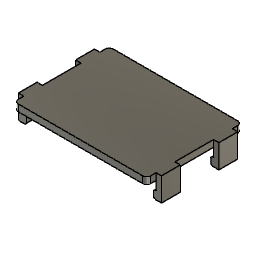
bluetooth module box (Autodesk Fusion 360 design; units mm, degrees)
Autodesk Fusion 360 part; units mm, degrees
note: some values were not read from the file. Set by a fixed rule: which sketch regions a step uses.
sketch "Sketch1" plane through (0, 0, 0) normal (0, 0, 1) x (1, 0, 0) in component "bottom"
  line L0 (0, 0) -> (49.2, 0)
  line L1 (49.2, 0) -> (49.2, 38.3)
  line L2 (49.2, 38.3) -> (0, 38.3)
  line L3 (0, 38.3) -> (0, 0)
  dimension "d6" = 38.3
  dimension "d7" = 49.2
  constraint horizontal L0
  constraint vertical L1
  constraint horizontal L2
  constraint vertical L3
  constraint coincident L0.start L3.end
  measures "d6" distance of L0.end L1.end
  measures "d7" distance of L1.end L2.end
extrude "Extrude1" add sketch "Sketch1" along normal blind 3 makes body 1 in component "bottom"
sketch "Sketch2" plane through (0, 0, 3) normal (0, 0, 1) x (-1, 0, 0) in component "bottom"
  line L0 (0, -38.3) -> (0, 0)
  line L1 (0, 0) -> (-49.2, 0)
  line L2 (-49.2, 0) -> (-49.2, -38.3)
  line L3 (-49.2, -38.3) -> (0, -38.3)
  line L4 (-46.2, -3) -> (-46.2, -35.3)
  line L5 (-46.2, -35.3) -> (-3, -35.3)
  line L6 (-3, -35.3) -> (-3, -3)
  line L7 (-3, -3) -> (-46.2, -3)
extrude "Extrude2" add sketch "Sketch2" along normal blind 12.2 bodies 1 in component "bottom"
sketch "Sketch3" plane through (0, 0, 0) normal (0, -1, 0) x (1, 0, 0) in component "bottom"
  line L0 (0, 0) -> (49.2, 0)
  line L1 (49.2, 0) -> (49.2, 15.2)
  line L2 (49.2, 15.2) -> (0, 15.2)
  line L3 (0, 15.2) -> (0, 0)
  line L4 (29.1, 10.2) -> (44.1, 10.2)
  line L5 (44.1, 10.2) -> (44.1, 7.2)
  line L6 (44.1, 7.2) -> (29.1, 7.2)
  line L7 (29.1, 7.2) -> (29.1, 10.2)
  line L8 (19.6, 12.2) -> (26.1, 12.2)
  line L9 (26.1, 12.2) -> (26.1, 7.2)
  line L10 (26.1, 7.2) -> (19.6, 7.2)
  line L11 (19.6, 7.2) -> (19.6, 12.2)
  line L12 (7.1, 10.2) -> (16.1, 10.2)
  line L13 (16.1, 10.2) -> (16.1, 7.2)
  line L14 (16.1, 7.2) -> (7.1, 7.2)
  line L15 (7.1, 7.2) -> (7.1, 10.2)
  dimension "d13" = 5.1
  dimension "d14" = 7.2
  dimension "d15" = 3
  dimension "d16" = 15
  dimension "d17" = 23.1
  dimension "d18" = 6.5
  dimension "d20" = 7.1
  dimension "d21" = 9
  dimension "d22" = 3
  dimension "d44" = 5
  constraint horizontal L4
  constraint vertical L5
  constraint horizontal L6
  constraint vertical L7
  constraint vertical L9
  constraint horizontal L10
  constraint vertical L11
  constraint collinear L6 L10
  constraint horizontal L12
  constraint vertical L13
  constraint horizontal L14
  constraint vertical L15
  constraint collinear L10 L14
  measures "d13" distance of L1 L5
  measures "d14" distance of L0 L6
  measures "d15" distance of L4.end L5.end
  measures "d16" distance of L4.start L4.end
  measures "d17" distance of L1 L9
  measures "d18" distance of L8.start L8.end
  measures "d20" distance of L3 L15
  measures "d21" distance of L12.start L12.end
  measures "d22" distance of L12.start L14.end
  measures "d44" distance of L8 L10
extrude "Extrude3" cut sketch "Sketch3" against normal blind 3 contours L4 L5 L6 L7 | L8 L9 L10 L11 | L12 L13 L14 L15 bodies 1 in component "bottom"
sketch "Sketch4" plane through (0, 0, 3) normal (0, 0, 1) x (-1, 0, 0) in component "bottom"
  line L0 (-46.2, -3) -> (-46.2, -35.3)
  line L1 (-46.2, -35.3) -> (-3, -35.3)
  line L2 (-3, -35.3) -> (-3, -3)
  line L3 (-3, -3) -> (-46.2, -3)
  line L4 (-5, -5) -> (-44.2, -5) construction
  line L5 (-44.2, -5) -> (-44.2, -33.3) construction
  line L6 (-44.2, -33.3) -> (-5, -33.3) construction
  line L7 (-5, -33.3) -> (-5, -5) construction
  circle A0 centre (-5, -33.3) radius 2
  circle A1 centre (-44.2, -33.3) radius 2
  circle A2 centre (-44.2, -5) radius 2
  circle A3 centre (-5, -5) radius 2
  line L8 (-3, -6) -> (-46.2, -6)
  line L9 (-46.2, -6) -> (-46.2, -3)
  line L10 (-46.2, -3) -> (-3, -3)
  line L11 (-3, -3) -> (-3, -6)
  dimension "d25" = -2
  dimension "d26" = 4
  dimension "d27" = 4
  dimension "d28" = 4
  dimension "d29" = 4
  dimension "d78" = 3
  constraint coincident L6.end L7.start
  constraint coincident L5.end L6.start
  constraint coincident L4.end L5.start
  constraint coincident L4.start L7.end
  constraint horizontal L8
  constraint vertical L9
  constraint horizontal L10
  constraint vertical L11
  constraint collinear L2 L11
  constraint collinear L0 L9
  constraint collinear L3 L10
  measures "d26" diameter of A0
  measures "d27" diameter of A1
  measures "d28" diameter of A2
  measures "d29" diameter of A3
  measures "d78" distance of L8 L10
extrude "Extrude4" add sketch "Sketch4" along normal blind 3 contours A2 L8 | A2 L8 | A3 L8 | A1 | A3 L8 | A0 bodies 1 in component "bottom"
extrude "Extrude7" cut 1 faces at (22.9333, 0, 2.4) along direction (0, 1, 0) blind 3 on bodies 1 bodies 1 in component "bottom"
extrude "Extrude9" add sketch "Sketch4" along normal up to surface (3 mm away) contours L0 L3 A2 L9 L10 | L3 A2 A3 L8 L10 | L2 L3 A3 L10 L11 bodies 1 in component "bottom"
chamfer "Chamfer1" distance 2 angle 45 1 edges at (24.6, 6, 6) on bodies 1 in component "bottom"
fillet "Fillet1" radius 1.5 1 edges at (0, 3, 7.6) on bodies 1 in component "bottom"
fillet "Fillet2" radius 1.5 1 edges at (49.2, 3, 7.6) on bodies 1 in component "bottom"
fillet "Fillet3" radius 1.5 1 edges at (0, 38.3, 7.6) on bodies 1 in component "bottom"
fillet "Fillet4" radius 1.5 1 edges at (49.2, 38.3, 7.6) on bodies 1 in component "bottom"
sketch "Sketch5" plane through (0, 38.3, 0) normal (0, 1, 0) x (-1, 0, 0) in component "bottom"
  line L0 (-47.7, 15.2) -> (-47.7, 0)
  line L1 (-47.7, 0) -> (-1.5, 0)
  line L2 (-1.5, 0) -> (-1.5, 15.2)
  line L3 (-1.5, 15.2) -> (-47.7, 15.2)
  line L4 (-30.5, 18) -> (-7.5, 18)
  line L5 (-7.5, 18) -> (-7.5, 9)
  line L6 (-7.5, 9) -> (-30.5, 9)
  line L7 (-30.5, 9) -> (-30.5, 18)
  line L8 (-49.7, 12.2) -> (-48.2, 12.2)
  line L9 (-48.2, 12.2) -> (-48.2, 8.7)
  line L10 (-48.2, 8.7) -> (-49.7, 8.7)
  line L11 (-49.7, 8.7) -> (-49.7, 12.2)
  line L12 (-49.2, 0) -> (-49.2, 15.2)
  line L13 (0, 15.2) -> (0, 0)
  line L14 (-1, 12.2) -> (0.5, 12.2)
  line L15 (0.5, 12.2) -> (0.5, 8.7)
  line L16 (0.5, 8.7) -> (-1, 8.7)
  line L17 (-1, 8.7) -> (-1, 12.2)
  line L18 (-49.2, 15.2) -> (-49.2, 0)
  line L19 (0, 0) -> (0, 15.2)
  line L20 (-3, 6) -> (-7, 6)
  line L21 (-3, 6) -> (-5, 6)
  dimension "d45" = 6
  dimension "d46" = 23
  dimension "d47" = 9
  dimension "d60" = 3.5
  dimension "d61" = 3
  dimension "d62" = 1.5
  dimension "d64" = 1.5
  dimension "d65" = 3
  dimension "d66" = 3.5
  dimension "d83" = 1
  dimension "d84" = 1
  dimension "d213" = 9
  constraint horizontal L4
  constraint vertical L5
  constraint horizontal L6
  constraint vertical L7
  constraint horizontal L8
  constraint vertical L9
  constraint horizontal L10
  constraint vertical L11
  constraint horizontal L14
  constraint vertical L15
  constraint horizontal L16
  constraint vertical L17
  measures "d45" distance of L2 L5
  measures "d46" distance of L5 L7
  measures "d47" distance of L4.start L6.end
  measures "d60" distance of L8.start L10.end
  measures "d61" distance of L8 L12.end
  measures "d62" distance of L8.start L8.end
  measures "d64" distance of L15 L17
  measures "d65" distance of L13.start L14
  measures "d66" distance of L14 L16
  measures "d83" distance of L9 L18
  measures "d84" distance of L17 L19
  measures "d213" distance of L1 L6
extrude "Extrude5" cut sketch "Sketch5" against normal blind 3 contours L3 L4 L5 L7 | L3 L5 L6 L7 bodies 1 in component "bottom"
cylinder "CylinderPrimitive5" add diameter 1.5 height 1.5 placed x (1, 0, 0) y (0, 1, 0) z (0, 0, 1) at (5, 33.3, 6) bodies 1 in component "bottom"
cylinder "CylinderPrimitive8" add diameter 1.5 height 1.5 placed x (1, 0, 0) y (0, 1, 0) z (0, 0, 1) at (5, 5, 6) bodies 1 in component "bottom"
extrude "Extrude6" cut sketch "Sketch5" against normal through all contours L8 L10 L11 L12 L18 | L8 L9 L10 L12 L18 | L13 L14 L15 L16 L19 | L13 L14 L16 L17 L19 bodies 1 in component "bottom"
sketch "Sketch1 (2)" plane through (0, 0, 0) normal (0, 0, 1) x (1, 0, 0) in component "lid"
  line L0 (0, 0) -> (49.2, 0)
  line L1 (49.2, 0) -> (49.2, 35.3)
  line L2 (0, 35.3) -> (0, 0)
  line L3 (49.2, 35.3) -> (0, 35.3)
  dimension "d218" = 49.2
  dimension "d219" = 35.3
  constraint horizontal L3
  constraint vertical L1
  constraint horizontal L0
  constraint vertical L2
  constraint coincident L0.start L2.end
  measures "d218" distance of L1.end L2.start
  measures "d219" distance of L0.start L2.start
extrude "Extrude1'" add sketch "Sketch1 (2)" along normal blind 2.5 separate body makes body 2 in component "lid"
fillet "Fillet1'" radius 1.5 4 edges at (49.2, 0, 1.25) (49.2, 35.3, 1.25) (0, 35.3, 1.25) (0, 0, 1.25) on bodies 2 in component "lid"
sketch "Sketch2 (2)" plane through (49.2, 0, 0) normal (1, 0, 0) x (0, 1, 0) in component "lid"
  line L0 (33.8, 0) -> (33.8, 2.5)
  line L1 (33.8, 2.5) -> (1.5, 2.5)
  line L2 (1.5, 2.5) -> (1.5, 0)
  line L3 (1.5, 0) -> (33.8, 0)
  line L4 (3.5, 2.5) -> (10.5, 2.5)
  line L5 (10.5, 2.5) -> (10.5, 0)
  line L6 (10.5, 0) -> (3.5, 0)
  line L7 (3.5, 0) -> (3.5, 2.5)
  line L8 (24.8, 2.5) -> (31.8, 2.5)
  line L9 (31.8, 2.5) -> (31.8, 0)
  line L10 (31.8, 0) -> (24.8, 0)
  line L11 (24.8, 0) -> (24.8, 2.5)
  dimension "d224" = 2
  dimension "d225" = 7
  dimension "d226" = 2
  dimension "d227" = 7
  constraint horizontal L4
  constraint vertical L5
  constraint horizontal L6
  constraint vertical L7
  constraint collinear L3 L6
  constraint collinear L1 L4
  constraint horizontal L8
  constraint vertical L9
  constraint horizontal L10
  constraint vertical L11
  constraint collinear L1 L8
  constraint collinear L3 L10
  measures "d224" distance of L2 L7
  measures "d225" distance of L4.start L4.end
  measures "d226" distance of L0 L9
  measures "d227" distance of L8.start L8.end
sketch "Sketch3 (2)" plane through (0, 0, 0) normal (-1, 0, 0) x (0, -1, 0) in component "lid"
  line L0 (-1.5, 0) -> (-1.5, 2.5)
  line L1 (-1.5, 2.5) -> (-33.8, 2.5)
  line L2 (-33.8, 2.5) -> (-33.8, 0)
  line L3 (-33.8, 0) -> (-1.5, 0)
  line L4 (-31.8, 2.5) -> (-24.8, 2.5)
  line L5 (-24.8, 2.5) -> (-24.8, 0)
  line L6 (-24.8, 0) -> (-31.8, 0)
  line L7 (-31.8, 0) -> (-31.8, 2.5)
  line L8 (-10.5, 2.5) -> (-3.5, 2.5)
  line L9 (-3.5, 2.5) -> (-3.5, 0)
  line L10 (-3.5, 0) -> (-10.5, 0)
  line L11 (-10.5, 0) -> (-10.5, 2.5)
  line L12 (-31.8, 0) -> (-24.8, 0)
  line L13 (-24.8, 2.5) -> (-31.8, 2.5)
  dimension "d228" = 2
  dimension "d229" = 7
  dimension "d230" = 7
  dimension "d231" = 2
  constraint horizontal L4
  constraint vertical L5
  constraint horizontal L6
  constraint vertical L7
  constraint horizontal L8
  constraint vertical L9
  constraint horizontal L10
  constraint vertical L11
  constraint collinear L1 L8
  constraint collinear L3 L10
  constraint collinear L6 L12
  constraint collinear L4 L13
  measures "d228" distance of L2 L7
  measures "d229" distance of L4.start L4.end
  measures "d230" distance of L8.start L8.end
  measures "d231" distance of L0 L9
extrude "Extrude2'" add sketch "Sketch2 (2)" along normal blind 2 contours L1 L3 L8 L9 L10 L11 | L1 L3 L4 L5 L6 L7 bodies 2 in component "lid"
extrude "Extrude3'" add sketch "Sketch3 (2)" along normal blind 2 contours L1 L3 L8 L9 L10 L11 | L1 L3 L4 L5 L6 L7 L12 L13 bodies 2 in component "lid"
sketch "Sketch4 (2)" plane through (0, 0, 0) normal (0, 0, -1) x (1, 0, 0) in component "lid"
  arc A0 (1.5, 0) -> (0, -1.5) centre (1.5, -1.5) ccw
  line L0 (0, -1.5) -> (0, -3.5)
  line L1 (0, -3.5) -> (-2, -3.5)
  line L2 (-2, -3.5) -> (-2, -10.5)
  line L3 (-2, -10.5) -> (0, -10.5)
  line L4 (0, -10.5) -> (0, -24.8)
  line L5 (0, -24.8) -> (-2, -24.8)
  line L6 (-2, -24.8) -> (-2, -31.8)
  line L7 (-2, -31.8) -> (0, -31.8)
  line L8 (0, -31.8) -> (0, -33.8)
  arc A1 (0, -33.8) -> (1.5, -35.3) centre (1.5, -33.8) ccw
  line L9 (1.5, -35.3) -> (47.7, -35.3)
  arc A2 (47.7, -35.3) -> (49.2, -33.8) centre (47.7, -33.8) ccw
  line L10 (49.2, -33.8) -> (49.2, -31.8)
  line L11 (49.2, -31.8) -> (51.2, -31.8)
  line L12 (51.2, -31.8) -> (51.2, -24.8)
  line L13 (51.2, -24.8) -> (49.2, -24.8)
  line L14 (49.2, -24.8) -> (49.2, -10.5)
  line L15 (49.2, -10.5) -> (51.2, -10.5)
  line L16 (51.2, -10.5) -> (51.2, -3.5)
  line L17 (51.2, -3.5) -> (49.2, -3.5)
  line L18 (49.2, -3.5) -> (49.2, -1.5)
  arc A3 (49.2, -1.5) -> (47.7, 0) centre (47.7, -1.5) ccw
  line L19 (47.7, 0) -> (1.5, 0)
  line L20 (49.2, -24.8) -> (51.2, -24.8)
  line L21 (51.2, -24.8) -> (51.2, -31.8)
  line L22 (51.2, -31.8) -> (49.2, -31.8)
  line L23 (49.2, -31.8) -> (49.2, -24.8)
  line L24 (49.2, -3.5) -> (51.2, -3.5)
  line L25 (51.2, -3.5) -> (51.2, -10.5)
  line L26 (51.2, -10.5) -> (49.2, -10.5)
  line L27 (49.2, -10.5) -> (49.2, -3.5)
  line L28 (-2, -3.5) -> (0, -3.5)
  line L29 (0, -3.5) -> (0, -10.5)
  line L30 (0, -10.5) -> (-2, -10.5)
  line L31 (-2, -10.5) -> (-2, -3.5)
  line L32 (-2, -24.8) -> (0, -24.8)
  line L33 (0, -24.8) -> (0, -31.8)
  line L34 (0, -31.8) -> (-2, -31.8)
  line L35 (-2, -31.8) -> (-2, -24.8)
  constraint horizontal L20
  constraint vertical L21
  constraint horizontal L22
  constraint vertical L23
  constraint horizontal L24
  constraint vertical L25
  constraint horizontal L26
  constraint vertical L27
  constraint horizontal L28
  constraint vertical L29
  constraint horizontal L30
  constraint vertical L31
  constraint horizontal L32
  constraint vertical L33
  constraint horizontal L34
  constraint vertical L35
  constraint collinear L16 L25
  constraint collinear L17 L24
  constraint collinear L18 L27
  constraint collinear L15 L26
  constraint collinear L12 L21
  constraint collinear L13 L20
  constraint collinear L11 L22
  constraint collinear L14 L23
  constraint collinear L6 L35
  constraint collinear L5 L32
  constraint collinear L4 L33
  constraint collinear L7 L34
  constraint collinear L2 L31
  constraint collinear L1 L28
  constraint collinear L3 L30
  constraint collinear L4 L29
extrude "Extrude4'" add sketch "Sketch4 (2)" along normal blind 6.25 contours L1 L2 L3 L28 L29 L30 L31 | L15 L16 L17 L24 L25 L26 L27 | L5 L6 L7 L32 L33 L34 L35 | L11 L12 L13 L20 L21 L22 L23 bodies 2 in component "lid"
sketch "Sketch15" plane through (49.2, 0, 0) normal (-1, 0, 0) x (0, -1, 0)
  line L0 (-24.8, 0) -> (-31.8, 0)
  line L1 (-31.8, 0) -> (-31.8, -6.25)
  line L2 (-31.8, -6.25) -> (-24.8, -6.25)
  line L3 (-24.8, -6.25) -> (-24.8, 0)
  line L4 (-31.8, -3.25) -> (-24.8, -3.25)
  line L5 (-24.8, -3.25) -> (-24.8, -6.25)
  line L6 (-24.8, -6.25) -> (-31.8, -6.25)
  line L7 (-31.8, -6.25) -> (-31.8, -3.25)
  dimension "d238" = 3
  constraint horizontal L4
  constraint vertical L5
  constraint horizontal L6
  constraint vertical L7
  constraint collinear L2 L6
  constraint collinear L1 L7
  constraint collinear L3 L5
  measures "d238" distance of L4.end L2.end
sketch "Sketch16" plane through (49.2, 0, 0) normal (-1, 0, 0) x (0, -1, 0)
  line L0 (-3.5, 0) -> (-10.5, 0)
  line L1 (-10.5, 0) -> (-10.5, -6.25)
  line L2 (-10.5, -6.25) -> (-3.5, -6.25)
  line L3 (-3.5, -6.25) -> (-3.5, 0)
  line L4 (-10.5, -3.25) -> (-3.5, -3.25)
  line L5 (-3.5, -3.25) -> (-3.5, -6.25)
  line L6 (-3.5, -6.25) -> (-10.5, -6.25)
  line L7 (-10.5, -6.25) -> (-10.5, -3.25)
  dimension "d239" = 3
  constraint horizontal L4
  constraint vertical L5
  constraint horizontal L6
  constraint vertical L7
  constraint collinear L3 L5
  constraint collinear L1 L7
  constraint collinear L2 L6
  measures "d239" distance of L4.end L2.end
sketch "Sketch17" plane through (0, 0, 0) normal (1, 0, 0) x (0, 1, 0)
  line L0 (31.8, 0) -> (24.8, 0)
  line L1 (24.8, 0) -> (24.8, -6.25)
  line L2 (24.8, -6.25) -> (31.8, -6.25)
  line L3 (31.8, -6.25) -> (31.8, 0)
  line L4 (24.8, -3.25) -> (31.8, -3.25)
  line L5 (31.8, -3.25) -> (31.8, -6.25)
  line L6 (31.8, -6.25) -> (24.8, -6.25)
  line L7 (24.8, -6.25) -> (24.8, -3.25)
  dimension "d240" = 3
  constraint horizontal L4
  constraint vertical L5
  constraint horizontal L6
  constraint vertical L7
  constraint collinear L3 L5
  constraint collinear L1 L7
  constraint collinear L2 L6
  measures "d240" distance of L4.end L2.end
sketch "Sketch18" plane through (0, 0, 0) normal (1, 0, 0) x (0, 1, 0)
  line L0 (10.5, 0) -> (3.5, 0)
  line L1 (3.5, 0) -> (3.5, -6.25)
  line L2 (3.5, -6.25) -> (10.5, -6.25)
  line L3 (10.5, -6.25) -> (10.5, 0)
  line L4 (3.5, -3.25) -> (10.5, -3.25)
  line L5 (10.5, -3.25) -> (10.5, -6.25)
  line L6 (10.5, -6.25) -> (3.5, -6.25)
  line L7 (3.5, -6.25) -> (3.5, -3.25)
  dimension "d241" = 3
  constraint horizontal L4
  constraint vertical L5
  constraint horizontal L6
  constraint vertical L7
  constraint collinear L3 L5
  constraint collinear L1 L7
  constraint collinear L2 L6
  measures "d241" distance of L4.end L2.end
extrude "Extrude5'" add sketch "Sketch15" sketch "Sketch16" along normal blind 1 contours L1 L2 L3 L4 L5 L6 L7 of sketch 2 contours L1 L2 L3 L4 L5 L6 L7 bodies 2 in component "lid"
extrude "Extrude6'" add sketch "Sketch17" sketch "Sketch18" along normal blind 1 contours L1 L2 L3 L4 L5 L6 L7 of sketch 2 contours L1 L2 L3 L4 L5 L6 L7 bodies 2 in component "lid"
chamfer "Chamfer1'" distance 0.5 angle 45 8 edges at (48.2, 28.3, -3.25) (48.2, 28.3, -6.25) (48.2, 7, -3.25) (48.2, 7, -6.25) (1, 7, -3.25) (1, 7, -6.25) (1, 28.3, -3.25) (1, 28.3, -6.25) on bodies 2 in component "lid"
move_body "Move1" bodies 1 to x (-1, 0, 0) y (0, -1, 0) z (0, 0, 1) at (48.2, 40.3, 0) in component "bottom"
cylinder "CylinderPrimitive11" add diameter 1.5 height 1.5 placed x (1, 0, 0) y (0, 1, 0) z (0, 0, 1) at (4, 7, 6) separate body makes body 3 in component "bottom"
cylinder "CylinderPrimitive12" add diameter 1.5 height 1.5 placed x (1, 0, 0) y (0, 1, 0) z (0, 0, 1) at (4, 35.3, 6) separate body makes body 4 in component "bottom"
sketch "Sketch5 (2)" plane through (0, 0, 0) normal (0, 0, -1) x (1, 0, 0) in component "lid"
  line L0 (49.2, -31.8) -> (49.2, -24.8)
  line L1 (49.2, -24.8) -> (49.2, -10.5)
  line L2 (49.2, -10.5) -> (49.2, -3.5)
  line L3 (49.2, -3.5) -> (49.2, -1.5)
  arc A0 (49.2, -1.5) -> (47.7, 0) centre (47.7, -1.5) ccw
  line L4 (47.7, 0) -> (1.5, 0)
  arc A1 (1.5, 0) -> (0, -1.5) centre (1.5, -1.5) ccw
  line L5 (0, -1.5) -> (0, -3.5)
  line L6 (0, -3.5) -> (0, -10.5)
  line L7 (0, -10.5) -> (0, -24.8)
  line L8 (0, -24.8) -> (0, -31.8)
  line L9 (0, -31.8) -> (0, -33.8)
  arc A2 (0, -33.8) -> (1.5, -35.3) centre (1.5, -33.8) ccw
  line L10 (1.5, -35.3) -> (47.7, -35.3)
  arc A3 (47.7, -35.3) -> (49.2, -33.8) centre (47.7, -33.8) ccw
  line L11 (49.2, -33.8) -> (49.2, -31.8)
  line L12 (46.1, -35.3) -> (42.2, -35.3)
  line L13 (42.2, -35.3) -> (42.2, -32.3)
  line L14 (42.2, -32.3) -> (46.1, -32.3)
  line L15 (46.1, -32.3) -> (46.1, -35.3)
  line L16 (42.2, -35.3) -> (32.7, -35.3)
  line L17 (32.7, -35.3) -> (32.7, -32.3)
  line L18 (32.7, -32.3) -> (42.2, -32.3)
  line L19 (42.2, -32.3) -> (42.2, -35.3)
  line L20 (32.7, -35.3) -> (29.7, -35.3)
  line L21 (29.7, -35.3) -> (29.7, -32.3)
  line L22 (29.7, -32.3) -> (32.7, -32.3)
  line L23 (32.7, -32.3) -> (32.7, -35.3)
  line L24 (22.5, -35.3) -> (20.5, -35.3)
  line L25 (20.5, -35.3) -> (20.5, -32.3)
  line L26 (20.5, -32.3) -> (22.5, -32.3)
  line L27 (22.5, -32.3) -> (22.5, -35.3)
  line L28 (20.5, -35.3) -> (6, -35.3)
  line L29 (6, -35.3) -> (6, -32.3)
  line L30 (6, -32.3) -> (20.5, -32.3)
  line L31 (20.5, -32.3) -> (20.5, -35.3)
  line L32 (6, -35.3) -> (3.1, -35.3)
  line L33 (3.1, -35.3) -> (3.1, -32.3)
  line L34 (3.1, -32.3) -> (6, -32.3)
  line L35 (6, -32.3) -> (6, -35.3)
  line L36 (29.7, -35.3) -> (22.5, -35.3)
  line L37 (22.5, -35.3) -> (22.5, -32.3)
  line L38 (22.5, -32.3) -> (29.7, -32.3)
  line L39 (29.7, -32.3) -> (29.7, -35.3)
  line L40 (14, -6) -> (4, -6)
  line L41 (4, -6) -> (4, -3)
  line L42 (4, -3) -> (14, -3)
  line L43 (14, -3) -> (14, -6)
  dimension "d305" = 3.1
  dimension "d306" = 3
  dimension "d307" = 3.9
  dimension "d308" = 9.5
  dimension "d309" = 3
  dimension "d310" = 3.1
  dimension "d311" = 2.9
  dimension "d312" = 14.5
  dimension "d313" = 2
  dimension "d315" = 10
  dimension "d316" = 3
  dimension "d317" = 3
  dimension "d319" = 4
  constraint horizontal L12
  constraint vertical L13
  constraint horizontal L14
  constraint vertical L15
  constraint horizontal L16
  constraint vertical L17
  constraint horizontal L18
  constraint vertical L19
  constraint horizontal L20
  constraint vertical L21
  constraint horizontal L22
  constraint vertical L23
  constraint collinear L10 L12
  constraint collinear L10 L16
  constraint collinear L10 L20
  constraint collinear L17 L23
  constraint collinear L13 L19
  constraint collinear L14 L18
  constraint collinear L18 L22
  constraint horizontal L24
  constraint vertical L25
  constraint horizontal L26
  constraint vertical L27
  constraint horizontal L28
  constraint vertical L29
  constraint horizontal L30
  constraint vertical L31
  constraint horizontal L32
  constraint vertical L33
  constraint horizontal L34
  constraint vertical L35
  constraint horizontal L36
  constraint vertical L37
  constraint horizontal L38
  constraint vertical L39
  constraint collinear L10 L36
  constraint collinear L10 L24
  constraint collinear L10 L28
  constraint collinear L10 L32
  constraint collinear L29 L35
  constraint collinear L25 L31
  constraint collinear L27 L37
  constraint collinear L21 L39
  constraint collinear L22 L38
  constraint collinear L26 L38
  constraint collinear L26 L30
  constraint collinear L30 L34
  constraint horizontal L40
  constraint vertical L41
  constraint horizontal L42
  constraint vertical L43
  measures "d305" distance of L11 L15
  measures "d306" distance of L12 L14
  measures "d307" distance of L15 L19
  measures "d308" distance of L19 L23
  measures "d309" distance of L21 L23
  measures "d310" distance of L9 L33
  measures "d311" distance of L33 L35
  measures "d312" distance of L29 L31
  measures "d313" distance of L27 L31
  measures "d315" distance of L40.start L40.end
  measures "d316" distance of L4 L42
  measures "d317" distance of L40.end L41.end
  measures "d319" distance of L5 L41
extrude "Extrude12" add sketch "Sketch5 (2)" along normal blind 2 contours L40 L41 L42 L43 bodies 2 in component "lid"
extrude "Extrude13" add sketch "Sketch5 (2)" along normal blind 7.5 contours L10 L12 L13 L14 L15 L19 | L10 L17 L20 L21 L22 L23 L39 | L10 L24 L25 L26 L27 L31 L37 | L10 L29 L32 L33 L34 L35 bodies 2 in component "lid"
extrude "Extrude14" add sketch "Sketch5 (2)" along normal blind 5 contours L10 L13 L16 L17 L18 L19 L23 bodies 2 in component "lid"
extrude "Extrude15" add sketch "Sketch5 (2)" along normal blind 2.5 contours L10 L21 L27 L36 L37 L38 L39 bodies 2 in component "lid"
extrude "Extrude16" add sketch "Sketch5 (2)" along normal blind 4.5 contours L10 L25 L28 L29 L30 L31 L35 bodies 2 in component "lid"
chamfer "Chamfer2" distance 1.5 angle 45 1 edges at (20.5, 32.3, -6) on bodies 2 in component "lid"
chamfer "Chamfer2" distance 1.5 angle 45 1 edges at (6, 32.3, -6) on bodies 2 in component "lid"
component "bottom" placed x (1, 0, 0) y (0, 1, 0) z (0, 0, 1) at (0.284, -0.5603, -1.1095)
component "lid" placed x (1, 0, 0) y (0, 1, 0) z (0, 0, 1) at (-0.716, 1.4397, 14.0905)
equation "wall_thickness = 3 mm"
equation "width = 32.1 mm"
equation "length = 43 mm"
equation "height = 12 mm"
equation "tolerance = 0.1 mm"
equation "d6 = width + 2 * wall_thickness + 2 * tolerance"
equation "d7 = length + 2 * wall_thickness + 2 * tolerance"
equation "d8 = wall_thickness"
equation "d10 = -wall_thickness"
equation "d11 = height + 2 * tolerance"
equation "d13 = wall_thickness + tolerance + 2 mm"
equation "d14 = wall_thickness + 4.2 mm"
equation "d17 = wall_thickness + tolerance + 20 mm"
equation "d20 = wall_thickness + tolerance + 4 mm"
equation "d23 = -wall_thickness"
equation "d27 = d26"
equation "d28 = d26"
equation "d29 = d26"
equation "d34 = wall_thickness / 2"
equation "d35 = wall_thickness / 2"
equation "d48 = -wall_thickness"
equation "d64 = d62"
equation "d65 = d61"
equation "d66 = d60"
equation "d72 = -wall_thickness"
equation "d75 = wall_thickness / 2"
equation "d77 = wall_thickness / 2"
equation "d78 = wall_thickness"
equation "d84 = d83"
equation "lid_thickness = 2.5 mm"
equation "d220 = lid_thickness"
equation "d223 = wall_thickness / 2"
equation "d305 = wall_thickness + tolerance"
equation "d306 = wall_thickness"
equation "d307 = 4 mm - tolerance"
equation "d310 = wall_thickness + tolerance"
equation "d311 = 3 mm - tolerance"
equation "d316 = wall_thickness"
equation "d317 = wall_thickness"
equation "d319 = wall_thickness + 1 mm"
